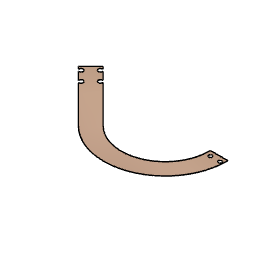
copper braid specimen curved v10 (Autodesk Fusion 360 design; units mm, degrees)
Autodesk Fusion 360 part; units mm, degrees
note: some values were not read from the file. Set by a fixed rule: which sketch regions a step uses; the direction of a hole.
sketch "Sketch1" plane through (0, 0, 0) normal (0, 1, 0) x (1, 0, 0)
  line L0 (18, 0) -> (0, 0)
  line L1 (-142.8787, 7.1213) -> (-130.1508, 19.8492)
  line L2 (0, 0) -> (-150, 0) construction
  line L3 (-150, 0) -> (-130.1508, 19.8492) construction
  line L4 (5, -5) -> (15, -5) construction
  line L5 (-136.5147, 13.4853) -> (-128.0294, 5) construction
  circle A0 centre (-128.0294, 5) radius 10 construction
  line L6 (-128.0294, 5) -> (-164.1172, -31.0878) construction
  line L7 (-128.0294, 5) -> (-128.0294, -5) construction
  line L8 (-130.1508, 19.8492) -> (-77.1177, -33.1838)
  line L9 (-142.8787, 7.1213) -> (-89.8457, -45.9117)
  line L10 (-77.1177, -33.1838) -> (-89.8457, -45.9117) construction
  line L11 (18, 0) -> (18, -1.2405)
  line L12 (0, 0) -> (0, -1.2405)
  line L13 (0, -1.2405) -> (18, -1.2405) construction
  arc A1 (-89.8457, -45.9117) -> (18, -1.2405) centre (-45.1745, -1.2405) ccw
  arc A2 (-77.1177, -33.1838) -> (0, -1.2405) centre (-45.1745, -1.2405) ccw
  point P0 (-128.0294, -5)
  point P1 (-118.0294, 5)
  point P2 (-128.0294, 15)
  point P3 (-138.0294, 5)
  dimension "d1" = 135
  dimension "d2" = 18
  dimension "d4" = 10
  dimension "d5" = 5
  dimension "d6" = 5
  dimension "d7" = 20
  dimension "d9" = 18
  dimension "d11" = 12
  dimension "d15" = 45
  dimension "d17" = 360
  dimension "d26" = 150
  dimension "d27" = 75
  dimension "d29" = 5
  constraint horizontal L0
  constraint parallel L0 L2
  constraint parallel L1 L3
  constraint coincident L0.end L2.start
  constraint horizontal L4
  constraint midpoint L1 L5.start
  constraint perpendicular L1 L5
  constraint coincident L5.end A0.centre
  constraint perpendicular L5 L6
  constraint coincident A0 P0
  constraint coincident P0 L7.end
  constraint perpendicular L1 L8
  constraint perpendicular L6 L9
  constraint perpendicular L8 L10
  constraint perpendicular L0 L11
  constraint perpendicular L0 L12
  constraint perpendicular L11 L13
  constraint tangent L9 A1
  constraint tangent L8 A2
  constraint tangent L12 A2
  measures "d1" angle of L2 L3
  measures "d2" distance of L0.start L0.end
  measures "d4" distance of L4.start L4.end
  measures "d5" distance of L0 L4
  measures "d6" horizontal distance of L0.end L4.start
  measures "d7" diameter of A0
  measures "d9" distance of L1.start L1.end
  measures "d11" distance of L5.start L5.end
  measures "d15" angle of L6 L7
  measures "d26" distance of L0.end L2.end
  measures "d27" distance of L1.start L9.end
  measures "d29" distance of L2 L5.end
extrude "Extrude1" add sketch "Sketch1" along normal blind 0.05
hole "Hole1" at (-128.0294, 0, -15) at (-138.0294, 0, -5) at (-128.0294, 0, 5) at (-118.0294, 0, -5) direction (0, 1, 0) diameter 4.5 depth 45 tip angle 118
hole "Hole2" at (5, 0, 5) at (15, 0, 5) direction (0, 1, 0) diameter 3.5 depth 45 tip angle 118
sketch "Sketch2" plane through (0, 0.05, 0) normal (0, 1, 0) x (-1, 0, 0)
  circle A0 centre (-5, 5) radius 1.75
  circle A1 centre (-15, 5) radius 1.75
  arc A2 (128.5743, 7.183) -> (130.2125, 5.5449) centre (128.0294, 5) ccw
  line L0 (128.5743, 7.183) -> (89.8457, 45.9117)
  arc A3 (89.8457, 45.9117) -> (-18, 1.2405) centre (45.1745, 1.2405) ccw
  line L1 (-18, 1.2405) -> (-18, 0)
  line L2 (-18, 0) -> (0, 0)
  line L3 (0, 0) -> (0, 1.2405)
  arc A4 (77.1177, 33.1838) -> (0, 1.2405) centre (45.1745, 1.2405) ccw
  line L4 (77.1177, 33.1838) -> (115.8464, -5.5449)
  arc A5 (117.4845, -7.183) -> (115.8464, -5.5449) centre (118.0294, -5) ccw
  line L5 (117.4845, -7.183) -> (125.8464, -15.5449)
  arc A6 (127.4845, -17.183) -> (125.8464, -15.5449) centre (128.0294, -15) ccw
  line L6 (127.4845, -17.183) -> (130.1508, -19.8492)
  line L7 (130.1508, -19.8492) -> (142.8787, -7.1213)
  line L8 (142.8787, -7.1213) -> (140.2125, -4.4551)
  arc A7 (138.5743, -2.817) -> (140.2125, -4.4551) centre (138.0294, -5) ccw
  line L9 (138.5743, -2.817) -> (130.2125, 5.5449)
